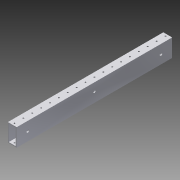
# Autodesk Inventor part: VersaFrame End Rail
Saved by Autodesk Inventor 2015 (Build 190159000, 159)
## iProperties
Created: 2014-12-18
Part Number: VersaFrame End Rail
Material: Aluminum 6061
Document SubType Name: Modeling
Designer: Nemo
Density: 2.7 g/cm^3
Appearance: Aluminum - Flat
Length: 17.500 in
HoleOffset: 0.500 in
Author: Nemo
Autodesk Inventor part; units mm, degrees
ref_plane "YZ Plane" through (0, 0, 0) normal (1, 0, 0) x (0, 1, 0)
ref_plane "XZ Plane" through (0, 0, 0) normal (0, 1, 0) x (-1, 0, 0)
ref_plane "XY Plane" through (0, 0, 0) normal (0, 0, 1) x (1, 0, 0)
sketch "Sketch1" plane through (0, 0, 0) normal (0, 0, 1) x (1, 0, 0)
  line L0 (12.7, -25.4) -> (-12.7, -25.4)
  line L1 (-12.7, -25.4) -> (-12.7, 25.4)
  line L2 (-12.7, 25.4) -> (12.7, 25.4)
  line L3 (12.7, 25.4) -> (12.7, -25.4)
  line L4 (12.7, -25.4) -> (-12.7, 25.4) construction
  line L5 (-12.7, -25.4) -> (12.7, 25.4) construction
  line L6 (10.16, 22.86) -> (-10.16, 22.86)
  line L7 (-10.16, 22.86) -> (-10.16, -22.86)
  line L8 (-10.16, -22.86) -> (10.16, -22.86)
  line L9 (10.16, -22.86) -> (10.16, 22.86)
  point P0 (0, 0)
  dimension "d0" = 25.4
  dimension "d1" = 50.8
  dimension "d2" = 2.54
  constraints: 20 end point, 4 parallel, 2 midpoint, 2 perpendicular, 1 horizontal, 3 other
  measures "d0" distance of L1.end L2.end
  measures "d1" distance of L0.end L1.end
  measures "d2" distance between parallel lines of L2 L6
extrude "Extrusion1" add sketch "Sketch1" along normal mid plane 444.5
sketch "Sketch2" plane through (-12.7, 25.4, 222.25) normal (0, 1, 0) x (1, 0, 0)
  point P0 (12.7, 222.25)
  point P1 (12.7, 234.95)
  point P2 (12.7, 209.55)
  dimension "HoleOffset" = 12.7
  dimension "d6" = 12.7
  constraints: 2 vertical alignment
  measures "HoleOffset" distance of point (12.7, 222.25) point (12.7, 234.95)
  measures "d6" distance of point (12.7, 222.25) point (12.7, 209.55)
hole "Hole1" at (0, 25.4, -12.7) at (0, 25.4, 12.7) direction (0, -1, 0) diameter 4.1656 end through all
pattern_linear "Rectangular Pattern1" count 31 spacing 50.8 along (0, 0, 1) of "Hole1" first direction both ways yes
sketch "Sketch3" plane through (12.7, -25.4, 222.25) normal (1, 0, 0) x (0, 0, -1)
  point P0 (222.25, 25.4)
  point P1 (31.75, 25.4)
  point P2 (412.75, 25.4)
  point P3 (222.25, 28.575)
  dimension "d18" = 190.5
  dimension "d19" = 190.5
  dimension "d27" = 3.175
  constraints: 2 horizontal alignment, 1 vertical alignment
  measures "d18" distance of point (412.75, 25.4) point (222.25, 25.4)
  measures "d19" distance of point (31.75, 25.4) point (222.25, 25.4)
  measures "d27" distance of point (222.25, 25.4) point (222.25, 28.575)
hole "Hole2" at (12.7, 0, 190.5) at (12.7, 0, -190.5) at (12.7, 3.175, 0) direction (-1, 0, 0) diameter 7.9375 end through all
equation "\"d19\" = d18"
body "Solid1"
